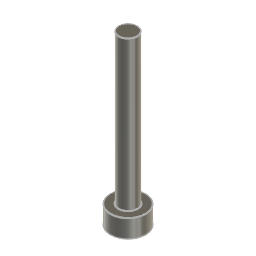
SNA (Autodesk Fusion 360 archive; units mm, degrees)
design "83.1215.02016"
Autodesk Fusion 360 part; units mm, degrees
sketch "Skizze1" plane through (0, 0, 0) normal (0, 0, 1) x (1, 0, 0)
  circle A0 centre (0, 0) radius 1
  circle A1 centre (0, 0) radius 1.9
  line L0 (1, 0.5774) -> (0, 1.1547)
  line L1 (0, 1.1547) -> (-1, 0.5774)
  line L2 (-1, 0.5774) -> (-1, -0.5774)
  line L3 (-1, -0.5774) -> (0, -1.1547)
  line L4 (0, -1.1547) -> (1, -0.5774)
  line L5 (1, -0.5774) -> (1, 0.5774)
  dimension "d1" = 2
  dimension "d2" = 3.8
  constraint coincident A0.centre A1.centre
  measures "d1" diameter of A0
  measures "d2" diameter of A1
extrude "Extrusion1" add sketch "Skizze1" along normal blind 2 contours A0 | A0 L4 L5 | A0 L0 L5 | A0 L0 L1 | A0 L3 L4 | A0 L1 L2 | A0 L2 L3 | A1
extrude "Extrusion2" add sketch "Skizze1" along normal blind 18 contours A0
extrude "Extrusion3" cut sketch "Skizze1" along normal blind 1 contours A0 | A0 L4 L5 | A0 L0 L5 | A0 L0 L1 | A0 L3 L4 | A0 L1 L2 | A0 L2 L3
fillet "Abrundung1" radius 0.05 4 faces at (-0.3333, 0.1925, 1) (-1.3, 0, 0) (1.5892, -0.1441, 2) (0.3412, -0.416, 18)
